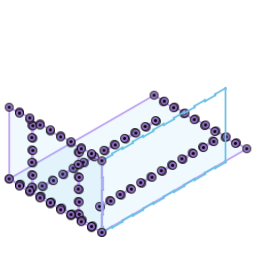
ventsulator (Autodesk Fusion 360 design; units mm, degrees)
Autodesk Fusion 360 part; units mm, degrees
sketch "Sketch1" plane through (0, 0, 0) normal (0, 0, 1) x (1, 0, 0)
  line L0 (-114.1021, 73.8944) -> (145.8979, 73.8944)
  line L1 (145.8979, 73.8944) -> (145.8979, -332.5056)
  line L2 (145.8979, -332.5056) -> (-114.1021, -332.5056)
  line L3 (-114.1021, -332.5056) -> (-114.1021, 73.8944)
  line L4 (15.8979, -332.5056) -> (15.8979, 73.8944) construction
  line L5 (-85.2132, -332.5056) -> (-85.2132, -329.5056)
  line L6 (-85.2132, -329.5056) -> (-56.3243, -329.5056)
  line L7 (-56.3243, -329.5056) -> (-56.3243, -332.5056)
  line L8 (-27.4354, -332.5056) -> (-27.4354, -329.5056)
  line L9 (-27.4354, -329.5056) -> (1.4535, -329.5056)
  line L10 (1.4535, -329.5056) -> (1.4535, -332.5056)
  line L11 (117.009, -332.5056) -> (117.009, -329.5056)
  line L12 (117.009, -329.5056) -> (88.1201, -329.5056)
  line L13 (88.1201, -329.5056) -> (88.1201, -332.5056)
  line L14 (59.2312, -332.5056) -> (59.2312, -329.5056)
  line L15 (59.2312, -329.5056) -> (30.3423, -329.5056)
  line L16 (30.3423, -329.5056) -> (30.3423, -332.5056)
  line L17 (-114.1021, -129.3056) -> (145.8979, -129.3056) construction
  line L18 (59.2312, 70.8944) -> (30.3423, 70.8944)
  line L19 (117.009, 73.8944) -> (117.009, 70.8944)
  line L20 (117.009, 70.8944) -> (88.1201, 70.8944)
  line L21 (88.1201, 70.8944) -> (88.1201, 73.8944)
  line L22 (59.2312, 73.8944) -> (59.2312, 70.8944)
  line L23 (30.3423, 70.8944) -> (30.3423, 73.8944)
  line L24 (-27.4354, 70.8944) -> (1.4535, 70.8944)
  line L25 (1.4535, 70.8944) -> (1.4535, 73.8944)
  line L26 (-27.4354, 73.8944) -> (-27.4354, 70.8944)
  line L27 (-56.3243, 70.8944) -> (-56.3243, 73.8944)
  line L28 (-85.2132, 70.8944) -> (-56.3243, 70.8944)
  line L29 (-85.2132, 73.8944) -> (-85.2132, 70.8944)
  line L30 (-47.6021, -303.6167) -> (-50.6021, -303.6167)
  line L31 (-50.6021, -303.6167) -> (-50.6021, -274.7278)
  line L32 (-50.6021, -274.7278) -> (-47.6021, -274.7278)
  line L33 (-47.6021, -274.7278) -> (-47.6021, -303.6167)
  line L34 (-47.6021, -303.6167) -> (-50.6021, -274.7278) construction
  line L35 (-50.6021, -303.6167) -> (-47.6021, -274.7278) construction
  line L36 (-114.1021, -260.2834) -> (145.8979, -260.2834) construction
  line L37 (-47.6021, -216.9501) -> (-50.6021, -245.8389) construction
  line L38 (-50.6021, -245.8389) -> (-47.6021, -245.8389)
  line L39 (-50.6021, -216.9501) -> (-50.6021, -245.8389)
  line L40 (-47.6021, -216.9501) -> (-50.6021, -216.9501)
  line L41 (-50.6021, -216.9501) -> (-47.6021, -245.8389) construction
  line L42 (-47.6021, -245.8389) -> (-47.6021, -216.9501)
  line L43 (-114.1021, -202.5056) -> (145.8979, -202.5056) construction
  line L44 (-50.6021, -188.0612) -> (-47.6021, -159.1723) construction
  line L45 (-50.6021, -130.2834) -> (-47.6021, -130.2834)
  line L46 (-47.6021, -130.2834) -> (-47.6021, -101.3945)
  line L47 (-47.6021, -188.0612) -> (-50.6021, -188.0612)
  line L48 (-50.6021, -188.0612) -> (-50.6021, -159.1723)
  line L49 (-47.6021, -188.0612) -> (-50.6021, -159.1723) construction
  line L50 (-50.6021, -159.1723) -> (-47.6021, -159.1723)
  line L51 (-50.6021, -101.3945) -> (-50.6021, -130.2834)
  line L52 (-50.6021, -101.3945) -> (-47.6021, -130.2834) construction
  line L53 (-47.6021, -101.3945) -> (-50.6021, -101.3945)
  line L54 (-47.6021, -159.1723) -> (-47.6021, -188.0612)
  line L55 (-47.6021, -101.3945) -> (-50.6021, -130.2834) construction
  line L56 (-114.1021, -86.9501) -> (145.8979, -86.9501) construction
  line L57 (-47.6021, 14.1611) -> (-50.6021, 14.1611)
  line L58 (-50.6021, -14.7278) -> (-47.6021, -14.7278)
  line L59 (-50.6021, 14.1611) -> (-50.6021, -14.7278)
  line L60 (-47.6021, -14.7278) -> (-47.6021, 14.1611)
  line L61 (-50.6021, 14.1611) -> (-47.6021, -14.7278) construction
  line L62 (-47.6021, 14.1611) -> (-50.6021, -14.7278) construction
  line L63 (-50.6021, -43.6167) -> (-47.6021, -43.6167)
  line L64 (-50.6021, -72.5056) -> (-47.6021, -43.6167) construction
  line L65 (-47.6021, -72.5056) -> (-50.6021, -43.6167) construction
  line L66 (-50.6021, -72.5056) -> (-50.6021, -43.6167)
  line L67 (-47.6021, -72.5056) -> (-50.6021, -72.5056)
  line L68 (-47.6021, -43.6167) -> (-47.6021, -72.5056)
  line L69 (15.8979, -332.5056) -> (15.8979, 73.8944) construction
  line L70 (79.3979, 16.1166) -> (82.3979, 16.1166)
  line L71 (82.3979, 16.1166) -> (82.3979, 45.0055)
  line L72 (82.3979, 45.0055) -> (79.3979, 45.0055)
  line L73 (79.3979, 45.0055) -> (79.3979, 16.1166)
  line L74 (79.3979, 16.1166) -> (82.3979, 45.0055) construction
  line L75 (82.3979, 16.1166) -> (79.3979, 45.0055) construction
  line L76 (145.8979, 1.6722) -> (-114.1021, 1.6722) construction
  line L77 (82.3979, -41.6612) -> (79.3979, -41.6612)
  line L78 (79.3979, -12.7723) -> (82.3979, -12.7723)
  line L79 (79.3979, -41.6612) -> (79.3979, -12.7723)
  line L80 (79.3979, -12.7723) -> (82.3979, -41.6612) construction
  line L81 (82.3979, -12.7723) -> (79.3979, -41.6612) construction
  line L82 (82.3979, -12.7723) -> (82.3979, -41.6612)
  line L83 (145.8979, -56.1056) -> (-114.1021, -56.1056) construction
  line L84 (79.3979, -128.3278) -> (82.3979, -128.3278)
  line L85 (82.3979, -128.3278) -> (82.3979, -157.2167)
  line L86 (82.3979, -157.2167) -> (79.3979, -157.2167)
  line L87 (79.3979, -128.3278) -> (82.3979, -157.2167) construction
  line L88 (82.3979, -128.3278) -> (79.3979, -157.2167) construction
  line L89 (79.3979, -157.2167) -> (79.3979, -128.3278)
  line L90 (82.3979, -70.5501) -> (79.3979, -70.5501)
  line L91 (82.3979, -99.4389) -> (79.3979, -70.5501) construction
  line L92 (79.3979, -70.5501) -> (79.3979, -99.4389)
  line L93 (82.3979, -99.4389) -> (82.3979, -70.5501)
  line L94 (79.3979, -99.4389) -> (82.3979, -99.4389)
  line L95 (79.3979, -99.4389) -> (82.3979, -70.5501) construction
  line L96 (145.8979, -171.6612) -> (-114.1021, -171.6612) construction
  line L97 (79.3979, -214.9945) -> (82.3979, -186.1056) construction
  line L98 (79.3979, -186.1056) -> (79.3979, -214.9945)
  line L99 (82.3979, -214.9945) -> (82.3979, -186.1056)
  line L100 (79.3979, -214.9945) -> (82.3979, -214.9945)
  line L101 (82.3979, -214.9945) -> (79.3979, -186.1056) construction
  line L102 (82.3979, -186.1056) -> (79.3979, -186.1056)
  line L103 (82.3979, -272.7723) -> (79.3979, -272.7723)
  line L104 (79.3979, -243.8834) -> (82.3979, -243.8834)
  line L105 (79.3979, -272.7723) -> (79.3979, -243.8834)
  line L106 (79.3979, -243.8834) -> (82.3979, -272.7723) construction
  line L107 (82.3979, -243.8834) -> (79.3979, -272.7723) construction
  line L108 (82.3979, -243.8834) -> (82.3979, -272.7723)
  point P0 (-49.1021, -289.1723)
  point P1 (-49.1021, -231.3945)
  point P2 (-49.1021, -115.8389)
  point P3 (-49.1021, -173.6167)
  point P4 (-49.1021, -0.2834)
  point P5 (-49.1021, -58.0612)
  point P6 (80.8979, 30.5611)
  point P7 (80.8979, -27.2167)
  point P8 (80.8979, -142.7723)
  point P9 (80.8979, -84.9945)
  point P10 (80.8979, -200.5501)
  point P11 (80.8979, -258.3278)
  dimension "d4" = 260
  dimension "d5" = 406.4
  dimension "d7" = 3
  dimension "d9" = 28.8889
  dimension "d10" = 28.8889
  dimension "d11" = 3
  dimension "d12" = 28.8889
  dimension "d13" = 28.8889
  dimension "d16" = 3
  dimension "d17" = 65
  dimension "d19" = 28.8889
  dimension "d20" = 28.8889
  dimension "d21" = 14.4444
  dimension "d22" = 28.8889
  dimension "d24" = 28.8889
  dimension "d25" = 3
  dimension "d26" = 28.8889
  dimension "d27" = 28.8889
  dimension "d28" = 28.8889
  dimension "d29" = 28.8889
  dimension "d30" = 28.8889
  dimension "d33" = 65
  constraint horizontal L0
  constraint vertical L1
  constraint horizontal L2
  constraint vertical L3
  constraint coincident L2 L4.start
  constraint coincident L0 L4.end
  constraint perpendicular L0 L4
  constraint midpoint L2 L4.start
  constraint coincident L2 L5.start
  constraint perpendicular L2 L5
  constraint perpendicular L5 L6
  constraint coincident L2 L7.end
  constraint perpendicular L2 L7
  constraint coincident L2 L8.start
  constraint perpendicular L2 L8
  constraint perpendicular L8 L9
  constraint coincident L2 L10.end
  constraint perpendicular L2 L10
  constraint symmetric L4 L5.start L11.start
  constraint symmetric L4 L5.end L11.end
  constraint symmetric L4 L6.end L12.end
  constraint symmetric L4 L7.end L13.end
  constraint symmetric L4 L8.start L14.start
  constraint symmetric L4 L8.end L14.end
  constraint symmetric L4 L9.end L15.end
  constraint symmetric L4 L10.end L16.end
  constraint coincident L3 L17.start
  constraint coincident L1 L17.end
  constraint perpendicular L1 L17
  constraint midpoint L1 L17.end
  constraint symmetric L5.start L17 L29.start
  constraint symmetric L5.end L17 L28.start
  constraint symmetric L6.end L17 L27.start
  constraint symmetric L7.end L17 L27.end
  constraint symmetric L8.start L17 L26.start
  constraint symmetric L8.end L17 L24.start
  constraint symmetric L9.end L17 L24.end
  constraint symmetric L10.end L17 L25.end
  constraint symmetric L11.start L17 L19.start
  constraint symmetric L11.end L17 L19.end
  constraint symmetric L12.end L17 L20.end
  constraint symmetric L13.end L17 L21.end
  constraint symmetric L14.start L17 L22.start
  constraint symmetric L14.end L17 L18.start
  constraint symmetric L15.end L17 L18.end
  constraint symmetric L16.end L17 L23.end
  constraint horizontal L30
  constraint perpendicular L30 L31
  constraint parallel L30 L32
  constraint parallel L31 L33
  constraint coincident L34 P0
  constraint coincident L35 P0
  constraint coincident L3 L36.start
  constraint coincident L1 L36.end
  constraint perpendicular L1 L36
  constraint symmetric L30.start L36 L37.start
  constraint symmetric L30.end L36 L39.start
  constraint symmetric L31.end L36 L37.end
  constraint symmetric L32.end L36 L38.end
  constraint symmetric P0 L36 P1
  constraint coincident L3 L43.start
  constraint coincident L1 L43.end
  constraint perpendicular L1 L43
  constraint symmetric L30.start L43 L46.end
  constraint symmetric L30.end L43 L51.start
  constraint symmetric L31.end L43 L45.start
  constraint symmetric L32.end L43 L45.end
  constraint symmetric P0 L43 P2
  constraint symmetric L39.start L43 L44.start
  constraint symmetric L37.start L43 L47.start
  constraint symmetric L37.end L43 L48.end
  constraint symmetric L38.end L43 L44.end
  constraint symmetric P1 L43 P3
  constraint coincident L3 L56.start
  constraint coincident L1 L56.end
  constraint perpendicular L1 L56
  constraint symmetric L46.end L56 L65.start
  constraint symmetric L45.end L56 L63.end
  constraint symmetric L48.end L56 L58.start
  constraint symmetric L45.start L56 L63.start
  constraint symmetric L44.end L56 L58.end
  constraint symmetric P2 L56 P5
  constraint symmetric L44.start L56 L57.end
  constraint symmetric P3 L56 P4
  constraint symmetric L47.start L56 L57.start
  constraint symmetric L51.start L56 L64.start
  constraint symmetric L69.start L4 L4.start
  constraint symmetric L69.end L4 L4.end
  constraint horizontal L70
  constraint perpendicular L70 L71
  constraint parallel L70 L72
  constraint parallel L71 L73
  constraint coincident L74 P6
  constraint coincident L75 P6
  constraint coincident L1 L76.start
  constraint coincident L3 L76.end
  constraint perpendicular L3 L76
  constraint symmetric L70.start L76 L78.start
  constraint symmetric L70.end L76 L78.end
  constraint symmetric L71.end L76 L77.start
  constraint symmetric L72.end L76 L77.end
  constraint symmetric P6 L76 P7
  constraint coincident L1 L83.start
  constraint coincident L3 L83.end
  constraint perpendicular L3 L83
  constraint symmetric L70.start L83 L84.start
  constraint symmetric L70.end L83 L84.end
  constraint symmetric L71.end L83 L85.end
  constraint symmetric L72.end L83 L86.end
  constraint symmetric P6 L83 P8
  constraint symmetric L77.start L83 L90.start
  constraint symmetric P7 L83 P9
  constraint symmetric L77.end L83 L90.end
  constraint symmetric L78.end L83 L91.start
  constraint symmetric L78.start L83 L92.end
  constraint coincident L1 L96.start
  constraint coincident L3 L96.end
  constraint perpendicular L3 L96
  constraint symmetric L86.end L96 L98.start
  constraint symmetric L85.end L96 L97.end
  constraint symmetric P8 L96 P10
  constraint symmetric L84.end L96 L99.start
  constraint symmetric L84.start L96 L97.start
  constraint symmetric L91.start L96 L104.end
  constraint symmetric P9 L96 P11
  constraint symmetric L92.end L96 L104.start
  constraint symmetric L90.end L96 L103.end
  constraint symmetric L90.start L96 L103.start
  measures "d4" distance of L1.end L2.end
  measures "d5" distance of L0.start L2.end
  measures "d7" distance of L5.start L5.end
  measures "d9" distance of L5.end L6.end
  measures "d10" distance of L3 L5
  measures "d11" distance of L8.start L8.end
  measures "d12" distance of L8.end L9.end
  measures "d13" distance of L7 L8
  measures "d16" distance of L30.start L30.end
  measures "d17" distance of L3 P0
  measures "d19" distance of L2 L30
  measures "d20" distance of L30.start L32.end
  measures "d21" distance of L32 L36
  measures "d22" distance of P1 L43
  measures "d24" distance of P2 L56
  measures "d25" distance of L70.start L70.end
  measures "d26" distance of L0 L72
  measures "d27" distance of L70.start L72.end
  measures "d28" distance of P6 L76
  measures "d29" distance of P7 L83
  measures "d30" distance of P8 L96
  measures "d33" distance of L1 P6
extrude "Extrude2" add sketch "Sketch1" along normal blind 3 contours L0 L1 L2 L3 L5 L6 L7 L8 L9 L10 L11 L12 L13 L14 L15 L16 L18 L19 L20 L21 L22 L23 L24 L25 L26 L27 L28 L29 makes body 1
sketch "Sketch4" plane through (0, -332.5056, 0) normal (0, -1, 0) x (1, 0, 0)
  line L0 (-114.1021, 0) -> (-85.2132, 0)
  line L1 (-85.2132, 0) -> (-85.2132, 3)
  line L2 (-85.2132, 3) -> (-114.1021, 3)
  line L3 (-114.1021, 3) -> (-114.1021, 0)
  line L4 (-114.1021, 0) -> (145.8979, 0)
  line L5 (145.8979, 0) -> (145.8979, 180)
  line L6 (145.8979, 180) -> (-114.1021, 180)
  line L7 (-114.1021, 180) -> (-114.1021, 0)
  line L8 (-114.1021, 3) -> (-85.2132, 3)
  line L9 (-85.2132, 3) -> (-85.2132, 0)
  line L10 (-56.3243, 0) -> (-56.3243, 3)
  line L11 (-56.3243, 3) -> (-27.4354, 3)
  line L12 (-27.4354, 3) -> (-27.4354, 0)
  line L13 (1.4535, 0) -> (1.4535, 3)
  line L14 (1.4535, 3) -> (30.3423, 3)
  line L15 (30.3423, 3) -> (30.3423, 0)
  line L16 (15.8979, 180) -> (15.8979, 0) construction
  line L17 (145.8979, 3) -> (117.009, 3)
  line L18 (88.1201, 3) -> (59.2312, 3)
  line L19 (88.1201, 0) -> (88.1201, 3)
  line L20 (30.3423, 0) -> (30.3423, 3)
  line L21 (30.3423, 3) -> (1.4535, 3)
  line L22 (1.4535, 3) -> (1.4535, 0)
  line L23 (59.2312, 3) -> (59.2312, 0)
  line L24 (117.009, 3) -> (117.009, 0)
  line L25 (-114.1021, 90) -> (145.8979, 90) construction
  line L26 (-114.1021, 177) -> (-114.1021, 180)
  line L27 (-85.2132, 180) -> (-85.2132, 177)
  line L28 (-56.3243, 177) -> (-27.4354, 177)
  line L29 (30.3423, 177) -> (30.3423, 180)
  line L30 (-114.1021, 180) -> (-85.2132, 180)
  line L31 (-27.4354, 177) -> (-27.4354, 180)
  line L32 (88.1201, 177) -> (59.2312, 177)
  line L33 (-114.1021, 180) -> (145.8979, 180)
  line L34 (-85.2132, 177) -> (-85.2132, 180)
  line L35 (117.009, 177) -> (117.009, 180)
  line L36 (30.3423, 180) -> (30.3423, 177)
  line L37 (-114.1021, 177) -> (-85.2132, 177)
  line L38 (-56.3243, 180) -> (-56.3243, 177)
  line L39 (88.1201, 180) -> (88.1201, 177)
  line L40 (1.4535, 180) -> (1.4535, 177)
  line L41 (-85.2132, 177) -> (-114.1021, 177)
  line L42 (145.8979, 177) -> (117.009, 177)
  line L43 (30.3423, 177) -> (1.4535, 177)
  line L44 (1.4535, 177) -> (1.4535, 180)
  line L45 (1.4535, 177) -> (30.3423, 177)
  line L46 (59.2312, 177) -> (59.2312, 180)
  line L47 (-114.1021, 30) -> (15.8979, 30) construction
  line L48 (-47.6021, 15) -> (-50.6021, 15)
  line L49 (-50.6021, 15) -> (-50.6021, 45)
  line L50 (-50.6021, 45) -> (-47.6021, 45)
  line L51 (-47.6021, 45) -> (-47.6021, 15)
  line L52 (-47.6021, 15) -> (-50.6021, 45) construction
  line L53 (-50.6021, 15) -> (-47.6021, 45) construction
  line L54 (-114.1021, 60) -> (15.8979, 60) construction
  line L55 (-50.6021, 75) -> (-47.6021, 75)
  line L56 (-50.6021, 105) -> (-50.6021, 75)
  line L57 (-47.6021, 105) -> (-50.6021, 75) construction
  line L58 (-47.6021, 75) -> (-47.6021, 105)
  line L59 (-47.6021, 105) -> (-50.6021, 105)
  line L60 (-50.6021, 105) -> (-47.6021, 75) construction
  line L61 (-47.6021, 135) -> (-47.6021, 165)
  line L62 (-50.6021, 135) -> (-47.6021, 135)
  line L63 (-50.6021, 165) -> (-47.6021, 135) construction
  line L64 (-47.6021, 165) -> (-50.6021, 135) construction
  line L65 (-50.6021, 165) -> (-50.6021, 135)
  line L66 (-47.6021, 165) -> (-50.6021, 165)
  line L67 (79.3979, 105) -> (82.3979, 75) construction
  line L68 (82.3979, 45) -> (79.3979, 45)
  line L69 (79.3979, 15) -> (82.3979, 45) construction
  line L70 (79.3979, 15) -> (82.3979, 15)
  line L71 (79.3979, 165) -> (82.3979, 165)
  line L72 (82.3979, 15) -> (82.3979, 45)
  line L73 (82.3979, 135) -> (79.3979, 135)
  line L74 (79.3979, 165) -> (82.3979, 135) construction
  line L75 (82.3979, 105) -> (79.3979, 75) construction
  line L76 (82.3979, 15) -> (79.3979, 45) construction
  line L77 (82.3979, 165) -> (79.3979, 135) construction
  line L78 (79.3979, 45) -> (79.3979, 15)
  line L79 (82.3979, 75) -> (79.3979, 75)
  line L80 (79.3979, 135) -> (79.3979, 165)
  line L81 (79.3979, 105) -> (82.3979, 105)
  line L82 (79.3979, 75) -> (79.3979, 105)
  line L83 (82.3979, 165) -> (82.3979, 135)
  line L84 (82.3979, 105) -> (82.3979, 75)
  point P0 (117.009, 0)
  point P1 (59.2312, 0)
  point P2 (117.009, 180)
  point P3 (15.8979, 180)
  point P4 (59.2312, 180)
  point P5 (0, 180)
  point P6 (-49.1021, 30)
  point P7 (-49.1021, 90)
  point P8 (-49.1021, 150)
  point P9 (80.8979, 150)
  point P10 (80.8979, 90)
  point P11 (80.8979, 30)
  dimension "d34" = 260
  dimension "d35" = 3
  dimension "d36" = 28.8889
  dimension "d37" = 3
  dimension "d38" = 28.8889
  dimension "d39" = 3
  dimension "d40" = 28.8889
  dimension "d41" = 130
  dimension "d42" = 28.8889
  dimension "d43" = 28.8889
  dimension "d44" = 90
  dimension "d55" = 30
  dimension "d57" = 30
  dimension "d58" = 3
  dimension "d59" = 65
  dimension "d60" = 30
  constraint horizontal L4
  constraint vertical L5
  constraint horizontal L6
  constraint vertical L7
  constraint coincident L0.start L3.end
  constraint coincident L7 L2.end
  constraint perpendicular L7 L8
  constraint coincident L4 L0.end
  constraint perpendicular L4 L9
  constraint coincident L4 L10.start
  constraint perpendicular L4 L10
  constraint perpendicular L10 L11
  constraint coincident L4 L12.end
  constraint perpendicular L4 L12
  constraint coincident L4 L13.start
  constraint perpendicular L4 L13
  constraint perpendicular L13 L14
  constraint coincident L4 L15.end
  constraint perpendicular L4 L15
  constraint coincident L6 P3
  constraint coincident L4 L16.end
  constraint perpendicular L4 L16
  constraint symmetric L0.end L16 P0
  constraint symmetric L2.end L16 L17.start
  constraint symmetric L1.end L16 L17.end
  constraint symmetric L10.start L16 L19.start
  constraint symmetric L10.end L16 L18.start
  constraint symmetric L11.end L16 L18.end
  constraint symmetric L12.end L16 P1
  constraint symmetric L13.start L16 L15.end
  constraint symmetric L13.end L16 L14.end
  constraint symmetric L14.end L16 L13.end
  constraint symmetric L15.end L16 L13.start
  constraint coincident P1 L23.end
  constraint coincident P0 L24.end
  constraint midpoint L7 L25.start
  constraint midpoint L5 L25.end
  constraint symmetric origin L25 P5
  constraint symmetric L0.start L25 L6.end
  constraint symmetric L0.end L25 L27.start
  constraint symmetric L1.end L25 L27.end
  constraint symmetric L2.end L25 L26.start
  constraint symmetric L4.end L25 L5.end
  constraint symmetric L10.start L25 L38.start
  constraint symmetric L10.end L25 L28.start
  constraint symmetric L11.end L25 L28.end
  constraint symmetric L12.end L25 L31.end
  constraint symmetric L13.start L25 L40.start
  constraint symmetric L13.end L25 L40.end
  constraint symmetric L14.end L25 L29.start
  constraint symmetric L15.end L25 L29.end
  constraint symmetric L16.end L25 P3
  constraint symmetric P0 L25 P2
  constraint symmetric L18.start L25 L32.start
  constraint symmetric P1 L25 P4
  constraint symmetric L17.start L25 L42.start
  constraint symmetric L17.end L25 L35.start
  constraint symmetric L18.end L25 L32.end
  constraint symmetric L19.start L25 L39.start
  constraint coincident L7 L47.start
  constraint coincident L16 L47.end
  constraint perpendicular L16 L47
  constraint horizontal L48
  constraint perpendicular L48 L49
  constraint parallel L48 L50
  constraint parallel L49 L51
  constraint coincident L52 P6
  constraint coincident L53 P6
  constraint coincident L47 P6
  constraint coincident L7 L54.start
  constraint coincident L16 L54.end
  constraint perpendicular L16 L54
  constraint symmetric L48.start L54 L57.start
  constraint symmetric L48.end L54 L56.start
  constraint symmetric L49.end L54 L55.start
  constraint symmetric L50.end L54 L55.end
  constraint symmetric P6 L54 P7
  constraint symmetric L25 L48.start L61.end
  constraint symmetric L25 L48.end L63.start
  constraint symmetric L25 L49.end L62.start
  constraint symmetric L25 L50.end L61.start
  constraint symmetric L25 P6 P8
  constraint symmetric L16 L48.start L69.start
  constraint symmetric L16 L48.end L70.end
  constraint symmetric L16 L49.end L68.start
  constraint symmetric L16 L50.end L68.end
  constraint symmetric L16 P6 P11
  constraint symmetric L16 P7 P10
  constraint symmetric L16 L55.end L75.end
  constraint symmetric L16 L56.start L75.start
  constraint symmetric L16 L55.start L67.end
  constraint symmetric L16 L57.start L67.start
  constraint symmetric L16 L61.start L73.end
  constraint symmetric L16 P8 P9
  constraint symmetric L16 L63.start L71.end
  constraint symmetric L16 L61.end L71.start
  constraint symmetric L16 L62.start L73.start
  measures "d34" distance of L5.end L6.end
  measures "d35" distance of L4 L8
  measures "d36" distance of L2.end L1.end
  measures "d37" distance of L10.start L10.end
  measures "d38" distance of L10.end L11.end
  measures "d39" distance of L13.start L13.end
  measures "d40" distance of L13.end L14.end
  measures "d41" distance of L7 L16
  measures "d42" distance of L9 L10
  measures "d43" distance of L12 L13
  measures "d44" distance of L4 L25
  measures "d55" distance of L4 L47
  measures "d57" distance of L48.end L49.end
  measures "d58" distance of L49.end L50.end
  measures "d59" distance of L7 P6
  measures "d60" distance of L47 L54
extrude "Extrude4" add sketch "Sketch4" against normal blind 3 separate body contours L1 L2 L4 L5 L6 L7 L8 L9 L10 L11 L12 L13 L14 L15 L17 L18 L19 L20 L21 L22 L23 L24 L27 L28 L29 L31 L32 L33 L34 L35 L36 L37 L38 L39 L40 L41 L42 L43 L44 L45 L46 makes body 2
sketch "Sketch6" plane through (145.8979, 0, 0) normal (1, 0, 0) x (0, 1, 0)
  line L0 (73.8944, 0) -> (73.8944, 3)
  line L1 (-332.5056, 3) -> (-332.5056, 0)
  line L2 (42.2337, 90) -> (-332.5056, 90) construction
  line L3 (-332.5056, 105) -> (-329.5056, 105)
  line L4 (-329.5056, 75) -> (-332.5056, 75)
  line L5 (-332.5056, 120) -> (-129.3056, 120) construction
  line L6 (-329.5056, 165) -> (-332.5056, 165)
  line L7 (-332.5056, 135) -> (-329.5056, 135)
  line L8 (-332.5056, 45) -> (-329.5056, 45)
  line L9 (-329.5056, 15) -> (-332.5056, 15)
  line L10 (-303.6167, 0) -> (-303.6167, 3)
  line L11 (-274.7278, 3) -> (-274.7278, 0)
  line L12 (-260.2834, 0) -> (-260.2834, 90) construction
  line L13 (-245.8389, 3) -> (-245.8389, 0)
  line L14 (-216.9501, 0) -> (-216.9501, 3)
  line L15 (-202.5056, 0) -> (-202.5056, 90) construction
  line L16 (-101.3945, 0) -> (-101.3945, 3)
  line L17 (-159.1723, 3) -> (-159.1723, 0)
  line L18 (-188.0612, 0) -> (-188.0612, 3)
  line L19 (-130.2834, 3) -> (-130.2834, 0)
  line L20 (-86.9501, 90) -> (-86.9501, 0) construction
  line L21 (-72.5056, 0) -> (-72.5056, 3)
  line L22 (-14.7278, 3) -> (-14.7278, 0)
  line L23 (-43.6167, 3) -> (-43.6167, 0)
  line L24 (14.1611, 0) -> (14.1611, 3)
  line L25 (-332.5056, 90) -> (14.1614, 90) construction
  line L26 (-14.7278, 177) -> (-14.7278, 180)
  line L27 (14.1611, 180) -> (14.1611, 177)
  line L28 (-101.3945, 180) -> (-101.3945, 177)
  line L29 (-43.6167, 177) -> (-43.6167, 180)
  line L30 (-72.5056, 180) -> (-72.5056, 177)
  line L31 (-274.7278, 177) -> (-274.7278, 180)
  line L32 (-216.9501, 180) -> (-216.9501, 177)
  line L33 (-130.2834, 177) -> (-130.2834, 180)
  line L34 (-303.6167, 180) -> (-303.6167, 177)
  line L35 (-188.0612, 180) -> (-188.0612, 177)
  line L36 (-159.1723, 177) -> (-159.1723, 180)
  line L37 (-245.8389, 177) -> (-245.8389, 180)
  line L38 (14.1611, 180) -> (-14.7278, 180)
  line L39 (-14.7278, 177) -> (-43.6167, 177)
  line L40 (-43.6167, 180) -> (-72.5056, 180)
  line L41 (-72.5056, 177) -> (-101.3945, 177)
  line L42 (-101.3945, 180) -> (-130.2834, 180)
  line L43 (-130.2834, 177) -> (-159.1723, 177)
  line L44 (-159.1723, 180) -> (-188.0612, 180)
  line L45 (-188.0612, 177) -> (-216.9501, 177)
  line L46 (-216.9501, 180) -> (-245.8389, 180)
  line L47 (-245.8389, 177) -> (-274.7278, 177)
  line L48 (-274.7278, 180) -> (-303.6167, 180)
  line L49 (-303.6167, 177) -> (-329.5056, 177)
  line L50 (-329.5056, 177) -> (-329.5056, 165)
  line L51 (-332.5056, 165) -> (-332.5056, 135)
  line L52 (-329.5056, 135) -> (-329.5056, 105)
  line L53 (-332.5056, 105) -> (-332.5056, 75)
  line L54 (-329.5056, 75) -> (-329.5056, 45)
  line L55 (-332.5056, 45) -> (-332.5056, 15)
  line L56 (-303.6167, 3) -> (-329.5056, 3)
  line L57 (-329.5056, 15) -> (-329.5056, 3)
  line L58 (-303.6167, 0) -> (-274.7278, 0)
  line L59 (-274.7278, 3) -> (-245.8389, 3)
  line L60 (-245.8389, 0) -> (-216.9501, 0)
  line L61 (-216.9501, 3) -> (-188.0612, 3)
  line L62 (-188.0612, 0) -> (-159.1723, 0)
  line L63 (-159.1723, 3) -> (-130.2834, 3)
  line L64 (-130.2834, 0) -> (-101.196, 0)
  line L65 (-101.3945, 3) -> (-72.5056, 3)
  line L66 (-72.5056, 0) -> (-43.6167, 0)
  line L67 (-43.6167, 3) -> (-14.7278, 3)
  line L68 (-14.7278, 0) -> (14.1614, 0)
  line L69 (14.1611, 0) -> (14.1614, 180)
  point P0 (-144.7278, 0)
  point P1 (-29.1723, 0)
  point P2 (-44.5945, 0)
  point P3 (-29.1723, 180)
  point P4 (-86.9501, 180)
  point P5 (14.1614, 180)
  point P6 (0, 180)
  point P7 (-202.5056, 180)
  point P8 (-144.7278, 180)
  point P9 (-260.2834, 180)
  dimension "d66" = 30
  dimension "d67" = 15
  dimension "d68" = 3
  dimension "d70" = 30
  dimension "d75" = 28.8889
  dimension "d76" = 3
  dimension "d77" = 14.4444
  dimension "d78" = 14.4444
  dimension "d79" = 28.8889
  constraint symmetric L3.start L5 L7.start
  constraint symmetric L3.end L5 L7.end
  constraint symmetric L4.start L5 L6.start
  constraint symmetric L4.end L5 L6.end
  constraint symmetric L2 L7.end L8.end
  constraint symmetric L2 L6.start L9.start
  constraint symmetric L2 L6.end L9.end
  constraint symmetric L2 L7.start L8.start
  constraint coincident L2 L12.end
  constraint perpendicular L2 L12
  constraint symmetric L10.start L12 L14.start
  constraint symmetric L10.end L12 L14.end
  constraint symmetric L11.start L12 L13.start
  constraint symmetric L11.end L12 L13.end
  constraint coincident L2 L15.end
  constraint perpendicular L2 L15
  constraint symmetric L10.start L15 L16.start
  constraint symmetric L10.end L15 L16.end
  constraint symmetric L11.start L15 L19.start
  constraint symmetric L11.end L15 L19.end
  constraint symmetric L12.start L15 P0
  constraint symmetric L13.start L15 L17.start
  constraint symmetric L14.start L15 L18.start
  constraint symmetric L14.end L15 L18.end
  constraint symmetric L13.end L15 L17.end
  constraint coincident L2 L20.start
  constraint symmetric L18.end L20 L24.end
  constraint symmetric L19.start L20 L23.start
  constraint symmetric L18.start L20 L24.start
  constraint symmetric P0 L20 P1
  constraint symmetric L19.end L20 L23.end
  constraint symmetric L16.start L20 L21.start
  constraint symmetric L17.end L20 L22.end
  constraint symmetric L17.start L20 L22.start
  constraint symmetric L16.end L20 L21.end
  constraint symmetric origin L2 P6
  constraint symmetric L2 L68.end P5
  constraint symmetric L2 L10.start L34.start
  constraint symmetric L2 L10.end L34.end
  constraint symmetric L2 L11.start L31.start
  constraint symmetric L2 L11.end L31.end
  constraint symmetric L2 L12.start P9
  constraint symmetric L2 L13.start L37.start
  constraint symmetric L2 L14.start L32.start
  constraint symmetric L2 L14.end L32.end
  constraint symmetric L2 L13.end L37.end
  constraint symmetric L2 L15.start P7
  constraint symmetric L2 L18.end L35.end
  constraint symmetric L2 L19.start L33.start
  constraint symmetric L2 L18.start L35.start
  constraint symmetric L2 P0 P8
  constraint symmetric L2 L19.end L33.end
  constraint symmetric L2 L16.start L28.start
  constraint symmetric L2 L17.end L36.end
  constraint symmetric L2 L17.start L36.start
  constraint symmetric L2 L16.end L28.end
  constraint symmetric L2 L20.end P4
  constraint symmetric L2 L24.start L27.start
  constraint symmetric L2 L22.start L26.start
  constraint symmetric L2 L23.start L29.start
  constraint symmetric L2 L23.end L29.end
  constraint symmetric L2 L21.start L30.start
  constraint symmetric L2 L22.end L26.end
  constraint symmetric L2 L24.end L27.end
  constraint symmetric L2 P1 P3
  constraint symmetric L2 L21.end L30.end
  constraint perpendicular L26 L38
  constraint perpendicular L6 L50
  constraint perpendicular L7 L51
  constraint perpendicular L4 L53
  constraint perpendicular L8 L54
  constraint perpendicular L56 L57
  constraint coincident P5 L69.end
  measures "d66" distance of L3.end L4.start
  measures "d67" distance of L2 L3
  measures "d68" distance of L4.start L4.end
  measures "d70" distance of L2 L5
  measures "d75" distance of L10.end L11.start
  measures "d76" distance of L11.start L11.end
  measures "d77" distance of L11 L12
  measures "d78" distance of L16 L20
  measures "d79" distance of L14 L18
sketch "Sketch10" plane through (0, 0, 3) normal (0, 0, 1) x (-1, 0, 0)
  line L0 (-79.3979, 186.1056) -> (-82.3979, 186.1056)
  line L1 (-82.3979, 186.1056) -> (-82.3979, 214.9945)
  line L2 (-82.3979, 214.9945) -> (-79.3979, 214.9945)
  line L3 (-79.3979, 214.9945) -> (-79.3979, 186.1056)
  line L4 (47.6021, -14.1611) -> (47.6021, 14.7278)
  line L5 (47.6021, 14.7278) -> (50.6021, 14.7278)
  line L6 (50.6021, 14.7278) -> (50.6021, -14.1611)
  line L7 (50.6021, -14.1611) -> (47.6021, -14.1611)
  line L8 (50.6021, 274.7278) -> (47.6021, 274.7278)
  line L9 (47.6021, 274.7278) -> (47.6021, 303.6167)
  line L10 (47.6021, 303.6167) -> (50.6021, 303.6167)
  line L11 (50.6021, 303.6167) -> (50.6021, 274.7278)
  line L12 (-82.3979, 99.4389) -> (-79.3979, 99.4389)
  line L13 (-79.3979, 99.4389) -> (-79.3979, 70.5501)
  line L14 (-79.3979, 70.5501) -> (-82.3979, 70.5501)
  line L15 (-82.3979, 70.5501) -> (-82.3979, 99.4389)
  line L16 (50.6021, 43.6167) -> (47.6021, 43.6167)
  line L17 (47.6021, 43.6167) -> (47.6021, 72.5056)
  line L18 (47.6021, 72.5056) -> (50.6021, 72.5056)
  line L19 (50.6021, 72.5056) -> (50.6021, 43.6167)
  line L20 (-82.3979, 157.2167) -> (-79.3979, 157.2167)
  line L21 (-79.3979, 157.2167) -> (-79.3979, 128.3278)
  line L22 (-79.3979, 128.3278) -> (-82.3979, 128.3278)
  line L23 (-82.3979, 128.3278) -> (-82.3979, 157.2167)
  line L24 (-79.3979, -16.1166) -> (-79.3979, -45.0055)
  line L25 (-79.3979, -45.0055) -> (-82.3979, -45.0055)
  line L26 (-82.3979, -45.0055) -> (-82.3979, -16.1166)
  line L27 (-82.3979, -16.1166) -> (-79.3979, -16.1166)
  line L28 (50.6021, 159.1723) -> (47.6021, 159.1723)
  line L29 (47.6021, 159.1723) -> (47.6021, 188.0612)
  line L30 (47.6021, 188.0612) -> (50.6021, 188.0612)
  line L31 (50.6021, 188.0612) -> (50.6021, 159.1723)
  line L32 (-79.3979, 12.7723) -> (-82.3979, 12.7723)
  line L33 (-82.3979, 12.7723) -> (-82.3979, 41.6612)
  line L34 (-82.3979, 41.6612) -> (-79.3979, 41.6612)
  line L35 (-79.3979, 41.6612) -> (-79.3979, 12.7723)
  line L36 (-79.3979, 243.8834) -> (-82.3979, 243.8834)
  line L37 (-82.3979, 243.8834) -> (-82.3979, 272.7723)
  line L38 (-82.3979, 272.7723) -> (-79.3979, 272.7723)
  line L39 (-79.3979, 272.7723) -> (-79.3979, 243.8834)
  line L40 (47.6021, 216.9501) -> (47.6021, 245.8389)
  line L41 (47.6021, 245.8389) -> (50.6021, 245.8389)
  line L42 (50.6021, 245.8389) -> (50.6021, 216.9501)
  line L43 (50.6021, 216.9501) -> (47.6021, 216.9501)
  line L44 (50.6021, 101.3945) -> (47.6021, 101.3945)
  line L45 (47.6021, 101.3945) -> (47.6021, 130.2834)
  line L46 (47.6021, 130.2834) -> (50.6021, 130.2834)
  line L47 (50.6021, 130.2834) -> (50.6021, 101.3945)
  line L48 (85.2132, 332.5056) -> (85.2132, 329.5056)
  line L49 (85.2132, 329.5056) -> (56.3243, 329.5056)
  line L50 (56.3243, 329.5056) -> (56.3243, 332.5056)
  line L51 (56.3243, 332.5056) -> (27.4354, 332.5056)
  line L52 (27.4354, 332.5056) -> (27.4354, 329.5056)
  line L53 (27.4354, 329.5056) -> (-1.4535, 329.5056)
  line L54 (-1.4535, 329.5056) -> (-1.4535, 332.5056)
  line L55 (-1.4535, 332.5056) -> (-30.3423, 332.5056)
  line L56 (-30.3423, 332.5056) -> (-30.3423, 329.5056)
  line L57 (-30.3423, 329.5056) -> (-59.2312, 329.5056)
  line L58 (-59.2312, 329.5056) -> (-59.2312, 332.5056)
  line L59 (-59.2312, 332.5056) -> (-88.1201, 332.5056)
  line L60 (-88.1201, 332.5056) -> (-88.1201, 329.5056)
  line L61 (-88.1201, 329.5056) -> (-117.009, 329.5056)
  line L62 (-117.009, 329.5056) -> (-117.009, 332.5056)
  line L63 (-117.009, 332.5056) -> (-145.8979, 332.5056)
  line L64 (-145.8979, 332.5056) -> (-145.8979, -73.8944)
  line L65 (-145.8979, -73.8944) -> (-117.009, -73.8944)
  line L66 (-117.009, -73.8944) -> (-117.009, -70.8944)
  line L67 (-117.009, -70.8944) -> (-88.1201, -70.8944)
  line L68 (-88.1201, -70.8944) -> (-88.1201, -73.8944)
  line L69 (-88.1201, -73.8944) -> (-59.2312, -73.8944)
  line L70 (-59.2312, -73.8944) -> (-59.2312, -70.8944)
  line L71 (-59.2312, -70.8944) -> (-30.3423, -70.8944)
  line L72 (-30.3423, -70.8944) -> (-30.3423, -73.8944)
  line L73 (-30.3423, -73.8944) -> (-1.4535, -73.8944)
  line L74 (-1.4535, -73.8944) -> (-1.4535, -70.8944)
  line L75 (-1.4535, -70.8944) -> (27.4354, -70.8944)
  line L76 (27.4354, -70.8944) -> (27.4354, -73.8944)
  line L77 (27.4354, -73.8944) -> (56.3243, -73.8944)
  line L78 (56.3243, -73.8944) -> (56.3243, -70.8944)
  line L79 (56.3243, -70.8944) -> (85.2132, -70.8944)
  line L80 (85.2132, -70.8944) -> (85.2132, -73.8944)
  line L81 (85.2132, -73.8944) -> (114.1021, -73.8944)
  line L82 (114.1021, -73.8944) -> (114.1021, 332.5056)
  line L83 (114.1021, 332.5056) -> (85.2132, 332.5056)
sketch "Sketch12" plane through (0, -332.5056, 0) normal (0, -1, 0) x (1, 0, 0)
  line L0 (79.3979, 15) -> (79.3979, 45)
  line L1 (79.3979, 45) -> (82.3979, 45)
  line L2 (82.3979, 45) -> (82.3979, 15)
  line L3 (82.3979, 15) -> (79.3979, 15)
  line L4 (79.3979, 105) -> (82.3979, 105)
  line L5 (82.3979, 105) -> (82.3979, 75)
  line L6 (82.3979, 75) -> (79.3979, 75)
  line L7 (79.3979, 75) -> (79.3979, 105)
  line L8 (-50.6021, 165) -> (-47.6021, 165)
  line L9 (-47.6021, 165) -> (-47.6021, 135)
  line L10 (-47.6021, 135) -> (-50.6021, 135)
  line L11 (-50.6021, 135) -> (-50.6021, 165)
  line L12 (-50.6021, 105) -> (-47.6021, 105)
  line L13 (-47.6021, 105) -> (-47.6021, 75)
  line L14 (-47.6021, 75) -> (-50.6021, 75)
  line L15 (-50.6021, 75) -> (-50.6021, 105)
  line L16 (-50.6021, 45) -> (-47.6021, 45)
  line L17 (-47.6021, 45) -> (-47.6021, 15)
  line L18 (-47.6021, 15) -> (-50.6021, 15)
  line L19 (-50.6021, 15) -> (-50.6021, 45)
  line L20 (79.3979, 165) -> (82.3979, 165)
  line L21 (82.3979, 165) -> (82.3979, 135)
  line L22 (82.3979, 135) -> (79.3979, 135)
  line L23 (79.3979, 135) -> (79.3979, 165)
  line L24 (88.1201, 180) -> (88.1201, 177)
  line L25 (88.1201, 177) -> (59.2312, 177)
  line L26 (59.2312, 177) -> (59.2312, 180)
  line L27 (59.2312, 180) -> (30.3423, 180)
  line L28 (30.3423, 180) -> (30.3423, 177)
  line L29 (30.3423, 177) -> (1.4535, 177)
  line L30 (1.4535, 177) -> (1.4535, 180)
  line L31 (1.4535, 180) -> (-27.4354, 180)
  line L32 (-27.4354, 180) -> (-27.4354, 177)
  line L33 (-27.4354, 177) -> (-56.3243, 177)
  line L34 (-56.3243, 177) -> (-56.3243, 180)
  line L35 (-56.3243, 180) -> (-85.2132, 180)
  line L36 (-85.2132, 180) -> (-85.2132, 177)
  line L37 (-85.2132, 177) -> (-114.1021, 177)
  line L38 (-114.1021, 177) -> (-114.1021, 3)
  line L39 (-114.1021, 3) -> (-85.2132, 3)
  line L40 (-85.2132, 3) -> (-85.2132, 0)
  line L41 (-85.2132, 0) -> (-56.3243, 0)
  line L42 (-56.3243, 0) -> (-56.3243, 3)
  line L43 (-56.3243, 3) -> (-27.4354, 3)
  line L44 (-27.4354, 3) -> (-27.4354, 0)
  line L45 (-27.4354, 0) -> (1.4535, 0)
  line L46 (1.4535, 0) -> (1.4535, 3)
  line L47 (1.4535, 3) -> (30.3423, 3)
  line L48 (30.3423, 3) -> (30.3423, 0)
  line L49 (30.3423, 0) -> (59.2312, 0)
  line L50 (59.2312, 0) -> (59.2312, 3)
  line L51 (59.2312, 3) -> (88.1201, 3)
  line L52 (88.1201, 3) -> (88.1201, 0)
  line L53 (88.1201, 0) -> (117.009, 0)
  line L54 (117.009, 0) -> (117.009, 3)
  line L55 (117.009, 3) -> (145.8979, 3)
  line L56 (145.8979, 3) -> (145.8979, 177)
  line L57 (145.8979, 177) -> (117.009, 177)
  line L58 (117.009, 177) -> (117.009, 180)
  line L59 (117.009, 180) -> (88.1201, 180)
hidden bodies 1 2
equation "boxlength = 406.4 mm"
equation "boxheight = 180 mm"
equation "boxwidth = 260 mm"
equation "d4 = boxwidth"
equation "d5 = boxlength"
equation "woodthickness = 3 mm"
equation "d7 = woodthickness"
equation "botfingerlength = ( boxwidth / 9 mm ) * 1 mm"
equation "d9 = botfingerlength"
equation "d10 = botfingerlength"
equation "d11 = woodthickness"
equation "d12 = botfingerlength"
equation "d13 = botfingerlength"
equation "d16 = woodthickness"
equation "d17 = boxwidth / 4"
equation "d19 = botfingerlength"
equation "d20 = botfingerlength"
equation "d21 = botfingerlength / 2"
equation "d22 = botfingerlength"
equation "d24 = botfingerlength"
equation "d25 = woodthickness"
equation "d26 = botfingerlength"
equation "d27 = botfingerlength"
equation "d28 = botfingerlength"
equation "d29 = botfingerlength"
equation "d30 = botfingerlength"
equation "d31 = woodthickness"
equation "d33 = boxwidth / 4"
equation "d34 = boxwidth"
equation "d35 = woodthickness"
equation "d36 = botfingerlength"
equation "d37 = woodthickness"
equation "d38 = botfingerlength"
equation "d39 = woodthickness"
equation "d40 = botfingerlength"
equation "d41 = boxwidth / 2"
equation "d42 = botfingerlength"
equation "d43 = botfingerlength"
equation "d44 = boxheight / 2"
equation "d55 = sidefingerlength"
equation "sidefingerlength = boxheight / 6"
equation "d57 = sidefingerlength"
equation "d58 = woodthickness"
equation "d59 = boxwidth / 4"
equation "d60 = sidefingerlength"
equation "d61 = -woodthickness"
equation "d66 = sidefingerlength"
equation "d67 = sidefingerlength / 2"
equation "d68 = woodthickness"
equation "d70 = sidefingerlength"
equation "d75 = botfingerlength"
equation "d76 = woodthickness"
equation "d77 = botfingerlength / 2"
equation "d78 = botfingerlength / 2"
equation "d79 = botfingerlength"
